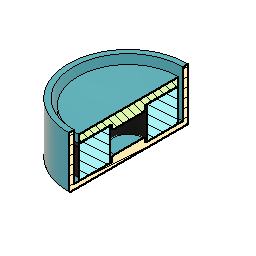
Sorbothane foot cups v3 (Autodesk Fusion 360 design; units mm, degrees)
Autodesk Fusion 360 part; units mm, degrees
note: some values were not read from the file. Set by a fixed rule: which face or edge a step refers to.
sketch "Base" plane through (0, 0, 0) normal (0, 1, 0) x (1, 0, 0)
  circle A0 centre (0, 0) radius 23
  circle A1 centre (0, 0) radius 6.5
  circle A2 centre (0, 0) radius 21
  dimension "d27" = 46
  dimension "d28" = 13
  dimension "d30" = 42
  constraint coincident A0.centre A1.centre
  measures "d27" diameter of A0
  measures "d28" diameter of A1
  measures "d30" diameter of A2
extrude "Extrude1" add sketch "Base" along normal blind 20 contours A0 | A1 | A2 makes body 1
shell "Shell1" thickness 2 removed faces 1 at (7.3261, 20, -8.1695) on bodies 1
extrude "Extrude2" add 1 faces at (7.1656, 2, -5.2255) along direction (0, 1, 0) blind 12.5 separate body on bodies 1 makes body 2
move_face "OffsetFaces1" offset -1.722 1 faces at (-20.8956, 6.1667, 2.0909) on bodies 2
hole "Hole1" at (0, 14.5, 0) direction (0, -1, 0) diameter 6.195 depth 13 tip angle 118 bodies 2
extrude "Extrude3" add 1 faces at (13.8098, 14.5, -1.0349) along direction (0, 1, 0) blind 3 separate body on bodies 2 makes body 3
move_body "Move1" bodies 3 to x (1, 0, 0) y (0, 1, 0) z (0, 0, 1) at (0, 21.174, 0)
sketch "Sketch2" plane through (0, 35.674, 0) normal (0, -1, 0) x (1, 0, 0)
  circle A0 centre (0, 0) radius 3.0975
  circle A1 centre (0, 0) radius 19.278
fillet "Fillet1" radius 1.242 2 edges at (-17.9734, 14.5, 6.9712) (-17.9734, 2, 6.9712) on bodies 2
extrude "Extrude7" add sketch "Base" against normal blind 5 from surface at 38.674 contours A1 bodies 3
extrude "Extrude6" add sketch "Base" along normal blind 4 contours A1 bodies 1
fillet "Fillet3" radius 0.95 2 edges at (-6.0601, 4, 2.3505) (-6.0601, 33.674, -2.3505) on bodies 1 3
move_face "OffsetFaces2" offset -3.948 1 faces at (0.3084, 6.1667, 3.0821) on bodies 2
move_body "Move2" bodies 3 to x (1, 0, 0) y (0, 1, 0) z (0, 0, 1) at (0, -21.0892, 0)
chamfer "Chamfer1" distance 0.3 angle 45 1 edges at (-21.4435, 0, 8.3172) on bodies 1
copy_body "Body->Comp1" bodies 1 removing the originals makes body 4 in component "Sorbothane Damper Base"
copy_body "Body->Comp2" bodies 2 removing the originals makes body 5 in component "Sorbothane Disc"
copy_body "Body->Comp3" bodies 3 removing the originals makes body 6 in component "Sorbothane Damper Top"
component "Sorbothane Damper Base" placed x (1, 0, 0) y (0, 1, 0) z (0, 0, 1) at (0, 0, 0)
component "Sorbothane Disc" placed x (1, 0, 0) y (0, 1, 0) z (0, 0, 1) at (0, 0, 0)
component "Sorbothane Damper Top" placed x (1, 0, 0) y (0, 1, 0) z (0, 0, 1) at (0, 0, 0)
named bodies: "Sorbothane Damper Base", "Sorbothane Disc", "Sorbothane Damper Top"
